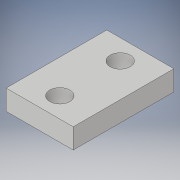
# Autodesk Inventor part: thumper-bumper-plunger-interface
Saved by Autodesk Inventor 2017 (Build 210142000, 142)
## iProperties
Created: 2017-02-27
Part Number: thumper-bumper-plunger-interface
Material: Generic
Document SubType Name: Modeling
Designer: John
Density: 1 g/cm^3
Appearance: Default
Author: John
Autodesk Inventor part; units mm, degrees
ref_plane "YZ Plane" through (0, 0, 0) normal (1, 0, 0) x (0, 1, 0)
ref_plane "XZ Plane" through (0, 0, 0) normal (0, 1, 0) x (-1, 0, 0)
ref_plane "XY Plane" through (0, 0, 0) normal (0, 0, 1) x (1, 0, 0)
sketch "Sketch1" plane through (0, 0, 0) normal (0, 1, 0) x (-1, 0, 0)
  line L0 (5, -7.5) -> (-5, -7.5)
  line L1 (-5, -7.5) -> (-5, 7.5)
  line L2 (-5, 7.5) -> (5, 7.5)
  line L3 (5, 7.5) -> (5, -7.5)
  line L4 (5, -7.5) -> (-5, 7.5) construction
  line L5 (-5, -7.5) -> (5, 7.5) construction
  circle A0 centre (0, -4.5) radius 1.5
  circle A1 centre (0, 4.5) radius 1.5
  line L6 (0, 4.5) -> (0, 7.5) construction
  line L7 (0, -7.5) -> (0, -4.5) construction
  point P0 (0, 0)
  dimension "d0" = 10
  dimension "d1" = 15
  dimension "d2" = 3
  dimension "d3" = 3
  dimension "d4" = 9
  dimension "d5" = 5
  dimension "d7" = 5
  constraints: 16 end point, 4 midpoint, 2 centre point, 2 parallel, 1 collinear, 1 horizontal, 1 perpendicular
  measures "d0" distance of L1.end L2.end
  measures "d1" distance of L0.end L1.end
  measures "d2" diameter of A0
  measures "d3" diameter of A1
  measures "d4" distance of L7.end L6.start
  measures "d5" distance from line of L6.start L3
  measures "d7" distance from line of L7.end L3
extrude "Extrusion1" add sketch "Sketch1" along normal blind 3
equation "\"d5\" = 0.5 * d0"
equation "\"d7\" = d5"
body "Solid1"
